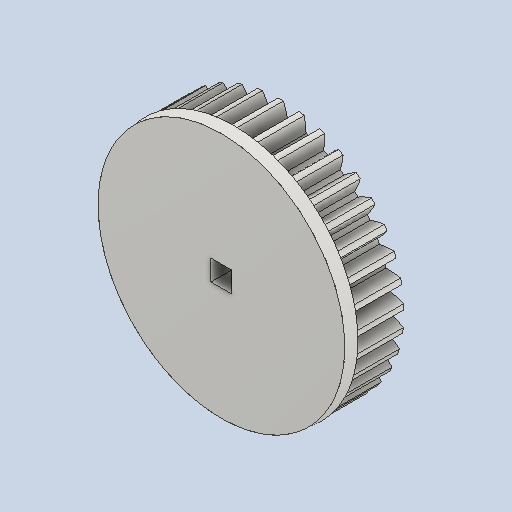
# Autodesk Inventor part: Spur Gear2
Saved by Autodesk Inventor 2022 (Build 260153000, 153)
## iProperties
CustomPartVersion: 1
Created: 2022-03-16
Part Number: Spur Gear2
Material: Steel
Document SubType Name: Modeling
Designer: zac-h
Categories: <?xml version="1.0" encoding="UTF-16"?> <MemberInstance><Categories><FamilyTemplate><FamilyTemplateParameter ValueType="xs:double" Id="1" ObjectReferenceKey="da_z" ObjectType="kUserParameterObject"/><FamilyTemplateParameter ValueType="xs:double" Id="2" ObjectReferenceKey="da_b" ObjectType="kUserParameterObject"/><FamilyTemplateParameter ValueType="xs:double" Id="3" ObjectReferenceKey="da_beta" ObjectType="kUserParameterObject"/><FamilyTemplateParameter ValueType="xs:double" Id="4" ObjectReferenceKey="da_da" ObjectType="kUserParameterObject"/><FamilyTemplateParameter ValueType="xs:double" Id="5" ObjectReferenceKey="da_aw" ObjectType="kUserParameterObject"/><FamilyTemplateParameter ValueType="xs:string" Id="6" ObjectReferenceKey="EAIAABAAAAC/AAAAAAAAAIAAAAAAAAAA" ObjectType="83910656" SubObjectId="SurfaceGeometry"/></FamilyTemplate><ParamToTemplateMap><ParamToTemplate CategoryParameter="//CategoryParameter[@InternalName='046C89C9-8512-4d59-83FE-43B91F4F132A']" TemplateParameter="1"/><ParamToTemplate CategoryParameter="//CategoryParameter[@InternalName='2552DF32-E462-4b46-AEBF-C6C7768E72AC']" TemplateParameter="2"/><ParamToTemplate CategoryParameter="//CategoryParameter[@InternalName='C9EE641D-15FC-4fae-A226-E94C4372FDD7']" TemplateParameter="3"/><ParamToTemplate><ParamToTemplate CategoryParameter="//CategoryParameter[@InternalName='00B6519A-459B-49c7-AD84-2E56D39A5744']" ConstantValue="0.273428"/></ParamToTemplate><ParamToTemplate><ParamToTemplate CategoryParameter="//CategoryParameter[@InternalName='04B31F0E-C7A6-4894-AA32-9629BEFACF47']" ConstantValue="1.000000"/></ParamToTemplate><ParamToTemplate><ParamToTemplate CategoryParameter="//CategoryParameter[@InternalName='43CBEC2E-7847-49e7-A936-2F7889FCB2D9']" ConstantValue="0.250000"/></ParamToTemplate><ParamToTemplate><ParamToTemplate CategoryParameter="//CategoryParameter[@InternalName='B1EFC894-105D-4ebd-86BF-FA20ED196853']" ConstantValue="0.333500"/></ParamToTemplate><ParamToTemplate><ParamToTemplate CategoryParameter="//CategoryParameter[@InternalName='51175063-3D10-4879-93E8-6246FE8B403D']" ConstantValue="2061532430.657340"/></ParamToTemplate><ParamToTemplate><ParamToTemplate CategoryParameter="//CategoryParameter[@InternalName='A3A52E27-4454-46a9-B0BD-C932399B70AF']" ConstantValue="0.300000"/></ParamToTemplate><ParamToTemplate><ParamToTemplate CategoryParameter="//CategoryParameter[@InternalName='91B76062-C214-41d9-B1B9-14D2AB99603D']" ConstantValue="0.100000"/></ParamToTemplate><ParamToTemplate><ParamToTemplate CategoryParameter="//CategoryParameter[@InternalName='374E806E-8B8A-4dda-A9AA-1039D6500AD2']" ConstantValue="10.000000"/></ParamToTemplate><ParamToTemplate><ParamToTemplate CategoryParameter="//CategoryParameter[@InternalName='2D373A89-B862-43d6-8D0B-0CBF12AB9F6C']" ConstantValue="0.253073"/></ParamToTemplate><ParamToTemplate CategoryParameter="//CategoryParameter[@InternalName='37777632-D6A2-4fac-9D53-DB8ACD95C989']" TemplateParameter="4"/><ParamToTemplate CategoryParameter="//CategoryParameter[@InternalName='FD1017F1-B727-4f7e-9707-0F86F1FF9423']" TemplateParameter="5"/><ParamToTemplate><ParamToTemplate CategoryParameter="//CategoryParameter[@InternalName='9E1B4470-B2D3-4ff1-B813-535BB4CDF51A']" ConstantValue="3523220.976809"/></ParamToTemplate><ParamToTemplate><ParamToTemplate CategoryParameter="//CategoryParameter[@InternalName='F8452263-BFF6-458c-9FB1-07C4B99E95CD']" ConstantValue="11397033.805607"/></ParamToTemplate><ParamToTemplate><ParamToTemplate CategoryParameter="//CategoryParameter[@InternalName='3E3BB259-FD49-497f-8171-6EBC954A3479']" ConstantValue="2.000000"/></ParamToTemplate><ParamToTemplate CategoryParameter="//CategoryParameter[@InternalName='27C3BAF2-7550-4e4b-AE2C-0DB134B7D9B7']" TemplateParameter="6"/></ParamToTemplateMap><Category DisplayName="Gear" InternalName="DC85795E-93AB-48d5-8EEE-5A27447B64BD" Mnemonic="Gear"><CategoryParameter DisplayName="z" InternalName="046C89C9-8512-4d59-83FE-43B91F4F132A" Mnemonic="z"/><CategoryParameter DisplayName="b" InternalName="2552DF32-E462-4b46-AEBF-C6C7768E72AC" Mnemonic="b"/><CategoryParameter DisplayName="||b|" InternalName="C9EE641D-15FC-4fae-A226-E94C4372FDD7" Mnemonic="beta"/><CategoryParameter DisplayName="x" InternalName="00B6519A-459B-49c7-AD84-2E56D39A5744" Mnemonic="x"/><CategoryParameter DisplayName="a*" InternalName="04B31F0E-C7A6-4894-AA32-9629BEFACF47" Mnemonic="a"/><CategoryParameter DisplayName="c*" InternalName="43CBEC2E-7847-49e7-A936-2F7889FCB2D9" Mnemonic="c"/><CategoryParameter DisplayName="r|.f|*" InternalName="B1EFC894-105D-4ebd-86BF-FA20ED196853" Mnemonic="rf"/><CategoryParameter DisplayName="E" InternalName="51175063-3D10-4879-93E8-6246FE8B403D" Mnemonic="E"/><CategoryParameter DisplayName="||m|" InternalName="A3A52E27-4454-46a9-B0BD-C932399B70AF" Mnemonic="mi"/><Category DisplayName="SpurGear" InternalName="26C5A22E-A91E-4dfd-A3B3-23CCAFAE1764" Mnemonic="SpurGear"><CategoryParameter DisplayName="m" InternalName="91B76062-C214-41d9-B1B9-14D2AB99603D" Mnemonic="m"/><CategoryParameter DisplayName="P" InternalName="374E806E-8B8A-4dda-A9AA-1039D6500AD2" Mnemonic="PP"/><CategoryParameter DisplayName="||a|" InternalName="2D373A89-B862-43d6-8D0B-0CBF12AB9F6C" Mnemonic="alpha"/><CategoryParameter DisplayName="d|.a|" InternalName="37777632-D6A2-4fac-9D53-DB8ACD95C989" Mnemonic="da"/><CategoryParameter DisplayName="a|.w|" InternalName="FD1017F1-B727-4f7e-9707-0F86F1FF9423" Mnemonic="aw"/><CategoryParameter DisplayName="||s||.Flim|" InternalName="9E1B4470-B2D3-4ff1-B813-535BB4CDF51A" Mnemonic="sFlim"/><CategoryParameter DisplayName="||s||.Hlim|" InternalName="F8452263-BFF6-458c-9FB1-07C4B99E95CD" Mnemonic="sHlim"/><CategoryParameter DisplayName="type" InternalName="3E3BB259-FD49-497f-8171-6EBC954A3479" Mnemonic="type"/><CategoryParameter DisplayName="PitchDiameter" InternalName="27C3BAF2-7550-4e4b-AE2C-0DB134B7D9B7" Mnemonic="IDS_PITCHDIAM"/></Category></Category></Categories></MemberInstance>
Density: 1 g/cm^3
Appearance: Steel
d9: 0.000 in
d14: 0.000 in
d15: 0.935 in
d16: 0.000 in
d17: 0.000 in
d18: 0.000 in
d19: 0.935 in
Author: zac-h
## iProperties of the stored document Spur Gear21_3DPrint.ipt
Created: 2022-03-19
Part Number: Spur Gear21_3DPrint
Material: Generic
Document SubType Name: Modeling
Designer: zac-h
Density: 1 g/cm^3
Appearance: Default
Author: zac-h
Autodesk Inventor part; units mm, degrees
sketch "Sketch1" plane through (0, 0, 0) normal (0, 0, 1) x (1, 0, 0)
  circle A0 centre (0, 0) radius 19.7541
  dimension "d0" = 39.5082
  constraints: 1 centre point
  measures "d0" diameter of A0
extrude "Extrusion1" add sketch "Sketch1" along normal blind 9.525
sketch "Sketch2" plane through (0, 0, 0) normal (0, 0, -1) x (-1, 0, 0)
  circle A0 centre (0, 0) radius 19.7541 projected
  circle A1 centre (0, 0) radius 18.5
  dimension "d3" = 37
  constraints: 1 centre point, 1 coincident
  measures "d3" diameter of A1
surface extrude "Pitch Diameter" sketch "Sketch2" against normal through all shown no curves A1
ref_plane "Work Plane1" through (0, 0, 0) normal (1, 0, 0) x (0, 1, 0)
ref_plane "Work Plane2" through (0, 0, 0) normal (0.9963975, 0.0848059, 0) x (0, 0, 1)
ref_plane "Work Plane3" through (0, 0, 4.7625) normal (0, 0, -1) x (-1, 0, 0)
spur gear teeth "Spur Gear" teeth 37 pitch diameter 37 tip diameter 39.5082 root diameter 35.0469 face width 9.525 start plane through (0, 0, 0) normal (0, 0, -1) x (-1, 0, 0)
sketch "Sketch3" plane through (0, 0, 9.525) normal (0, 0, 1) x (1, 0, 0)
  line L0 (-1.6625, 1.6625) -> (1.6625, 1.6625)
  line L1 (1.6625, 1.6625) -> (1.6625, -1.6625)
  line L2 (1.6625, -1.6625) -> (-1.6625, -1.6625)
  line L3 (-1.6625, -1.6625) -> (-1.6625, 1.6625)
  line L4 (-1.6625, 1.6625) -> (1.6625, -1.6625) construction
  line L5 (1.6625, 1.6625) -> (-1.6625, -1.6625) construction
  point P0 (0, 0)
  dimension "d20" = 3.325
  constraints: 12 end point, 2 midpoint, 2 parallel, 2 perpendicular, 1 horizontal
  measures "d20" distance of L1.end L2.end
extrude "Extrusion2" cut sketch "Sketch3" against normal through all
sketch "Sketch4" plane through (0, 0, 0) normal (0, 0, -1) x (-1, 0, 0)
  circle A0 centre (0, 0) radius 6.05
  line L0 (-1.6625, -1.6625) -> (-1.6625, 1.6625) projected
  line L1 (-1.6625, 1.6625) -> (1.6625, 1.6625) projected
  line L2 (1.6625, 1.6625) -> (1.6625, -1.6625) projected
  line L3 (1.6625, -1.6625) -> (-1.6625, -1.6625) projected
  arc A1 (4.0546, 17.0479) -> (3.751, 19.3947) centre (-6.6227, 16.8595) ccw projected
  arc A2 (3.751, 19.3947) -> (2.9244, 19.5364) centre (0, 0) ccw projected
  arc A3 (2.9244, 19.5364) -> (1.8564, 17.4248) centre (11.861, 13.6902) ccw projected
  arc A4 (1.8564, 17.4248) -> (1.1152, 17.4879) centre (0, 0) ccw projected
  arc A5 (1.1152, 17.4879) -> (0.4193, 19.7496) centre (-9.3767, 15.4978) ccw projected
  arc A6 (0.4193, 19.7496) -> (-0.4193, 19.7496) centre (0, 0) ccw projected
  arc A7 (-0.4193, 19.7496) -> (-1.1152, 17.4879) centre (9.3767, 15.4978) ccw projected
  arc A8 (-1.1152, 17.4879) -> (-1.8564, 17.4248) centre (0, 0) ccw projected
  arc A9 (-1.8564, 17.4248) -> (-2.9244, 19.5364) centre (-11.861, 13.6902) ccw projected
  arc A10 (-2.9244, 19.5364) -> (-3.751, 19.3947) centre (0, 0) ccw projected
  arc A11 (-3.751, 19.3947) -> (-4.0546, 17.0479) centre (6.6227, 16.8595) ccw projected
  arc A12 (-4.0546, 17.0479) -> (-4.7745, 16.8605) centre (0, 0) ccw projected
  arc A13 (-4.7745, 16.8605) -> (-6.1841, 18.7612) centre (-14.004, 11.4887) ccw projected
  arc A14 (-6.1841, 18.7612) -> (-6.9747, 18.4818) centre (0, 0) ccw projected
  arc A15 (-6.9747, 18.4818) -> (-6.8774, 16.1175) centre (3.6782, 17.7363) ccw projected
  arc A16 (-6.8774, 16.1175) -> (-7.5552, 15.811) centre (0, 0) ccw projected
  arc A17 (-7.5552, 15.811) -> (-9.2658, 17.4462) centre (-15.7442, 8.9568) ccw projected
  arc A18 (-9.2658, 17.4462) -> (-9.9978, 17.0372) centre (0, 0) ccw projected
  arc A19 (-9.9978, 17.0372) -> (-9.5023, 14.7233) centre (0.6278, 18.1028) ccw projected
  arc A20 (-9.5023, 14.7233) -> (-10.1186, 14.3068) centre (0, 0) ccw projected
  arc A21 (-10.1186, 14.3068) -> (-12.0809, 15.6293) centre (-17.0314, 6.1672) ccw projected
  arc A22 (-12.0809, 15.6293) -> (-12.7333, 15.1025) centre (0, 0) ccw projected
  arc A23 (-12.7333, 15.1025) -> (-11.8539, 12.9057) centre (-2.4406, 17.9485) ccw projected
  arc A24 (-11.8539, 12.9057) -> (-12.3909, 12.3909) centre (0, 0) ccw projected
  arc A25 (-12.3909, 12.3909) -> (-14.5485, 13.3628) centre (-17.8287, 3.2001) ccw projected
  arc A26 (-14.5485, 13.3628) -> (-15.1025, 12.7333) centre (0, 0) ccw projected
  arc A27 (-15.1025, 12.7333) -> (-13.8644, 10.7167) centre (-5.4388, 17.2778) ccw projected
  arc A28 (-13.8644, 10.7167) -> (-14.3068, 10.1186) centre (0, 0) ccw projected
  arc A29 (-14.3068, 10.1186) -> (-16.5975, 10.7119) centre (-18.1131, 0.141) ccw projected
  arc A30 (-16.5975, 10.7119) -> (-17.0372, 9.9978) centre (0, 0) ccw projected
  arc A31 (-17.0372, 9.9978) -> (-15.4761, 8.2195) centre (-8.2805, 16.1101) ccw projected
  arc A32 (-15.4761, 8.2195) -> (-15.811, 7.5552) centre (0, 0) ccw projected
  arc A33 (-15.811, 7.5552) -> (-18.1691, 7.7528) centre (-17.8764, -2.9221) ccw projected
  arc A34 (-18.1691, 7.7528) -> (-18.4818, 6.9747) centre (0, 0) ccw projected
  arc A35 (-18.4818, 6.9747) -> (-16.6426, 5.4857) centre (-10.884, 14.479) ccw projected
  arc A36 (-16.6426, 5.4857) -> (-16.8605, 4.7745) centre (0, 0) ccw projected
  arc A37 (-16.8605, 4.7745) -> (-19.218, 4.5707) centre (-17.1254, -5.9012) ccw projected
  arc A38 (-19.218, 4.5707) -> (-19.3947, 3.751) centre (0, 0) ccw projected
  arc A39 (-19.3947, 3.751) -> (-17.3303, 2.5942) centre (-13.1744, 12.4313) ccw projected
  arc A40 (-17.3303, 2.5942) -> (-17.4248, 1.8564) centre (0, 0) ccw projected
  arc A41 (-17.4248, 1.8564) -> (-19.714, 1.2571) centre (-15.8818, -8.7105) ccw projected
  arc A42 (-19.714, 1.2571) -> (-19.7496, 0.4193) centre (0, 0) ccw projected
  arc A43 (-19.7496, 0.4193) -> (-17.5195, -0.3719) centre (-15.0858, 10.026) ccw projected
  arc A44 (-17.5195, -0.3719) -> (-17.4879, -1.1152) centre (0, 0) ccw projected
  arc A45 (-17.4879, -1.1152) -> (-19.6429, -2.0927) centre (-14.1812, -11.2693) ccw projected
  arc A46 (-19.6429, -2.0927) -> (-19.5364, -2.9244) centre (0, 0) ccw projected
  arc A47 (-19.5364, -2.9244) -> (-17.2046, -3.3274) centre (-16.5633, 7.3323) ccw projected
  arc A48 (-17.2046, -3.3274) -> (-17.0479, -4.0546) centre (0, 0) ccw projected
  arc A49 (-17.0479, -4.0546) -> (-19.0067, -5.3822) centre (-12.0727, -13.5038) ccw projected
  arc A50 (-19.0067, -5.3822) -> (-18.7612, -6.1841) centre (0, 0) ccw projected
  arc A51 (-18.7612, -6.1841) -> (-16.3948, -6.1871) centre (-17.5642, 4.4276) ccw projected
  arc A52 (-16.3948, -6.1871) -> (-16.1175, -6.8774) centre (0, 0) ccw projected
  arc A53 (-16.1175, -6.8774) -> (-17.8237, -8.517) centre (-9.6169, -15.3499) ccw projected
  arc A54 (-17.8237, -8.517) -> (-17.4462, -9.2658) centre (0, 0) ccw projected
  arc A55 (-17.4462, -9.2658) -> (-15.1134, -8.8689) centre (-18.0598, 1.3956) ccw projected
  arc A56 (-15.1134, -8.8689) -> (-14.7233, -9.5023) centre (0, 0) ccw projected
  arc A57 (-14.7233, -9.5023) -> (-16.128, -11.4067) centre (-6.8844, -16.7543) ccw projected
  arc A58 (-16.128, -11.4067) -> (-15.6293, -12.0809) centre (0, 0) ccw projected
  arc A59 (-15.6293, -12.0809) -> (-13.3971, -11.2955) centre (-18.0359, -1.6766) ccw projected
  arc A60 (-13.3971, -11.2955) -> (-12.9057, -11.8539) centre (0, 0) ccw projected
  arc A61 (-12.9057, -11.8539) -> (-13.9682, -13.9682) centre (-3.9539, -17.6768) ccw projected
  arc A62 (-13.9682, -13.9682) -> (-13.3628, -14.5485) centre (0, 0) ccw projected
  arc A63 (-13.3628, -14.5485) -> (-11.2955, -13.3971) centre (-17.4931, -4.7006) ccw projected
  arc A64 (-11.2955, -13.3971) -> (-10.7167, -13.8644) centre (0, 0) ccw projected
  arc A65 (-10.7167, -13.8644) -> (-11.4067, -16.128) centre (-0.9097, -18.0908) ccw projected
  arc A66 (-11.4067, -16.128) -> (-10.7119, -16.5975) centre (0, 0) ccw projected
  arc A67 (-10.7119, -16.5975) -> (-8.8689, -15.1134) centre (-16.4471, -7.5893) ccw projected
  arc A68 (-8.8689, -15.1134) -> (-8.2195, -15.4761) centre (0, 0) ccw projected
  arc A69 (-8.2195, -15.4761) -> (-8.517, -17.8237) centre (2.1608, -17.9843) ccw projected
  arc A70 (-8.517, -17.8237) -> (-7.7528, -18.1691) centre (0, 0) ccw projected
  arc A71 (-7.7528, -18.1691) -> (-6.1871, -16.3948) centre (-14.9279, -10.2597) ccw projected
  arc A72 (-6.1871, -16.3948) -> (-5.4857, -16.6426) centre (0, 0) ccw projected
  arc A73 (-5.4857, -16.6426) -> (-5.3822, -19.0067) centre (5.1691, -17.3604) ccw projected
  arc A74 (-5.3822, -19.0067) -> (-4.5707, -19.218) centre (0, 0) ccw projected
  arc A75 (-4.5707, -19.218) -> (-3.3274, -17.2046) centre (-12.9793, -12.635) ccw projected
  arc A76 (-3.3274, -17.2046) -> (-2.5942, -17.3303) centre (0, 0) ccw projected
  arc A77 (-2.5942, -17.3303) -> (-2.0927, -19.6429) centre (8.0286, -16.2371) ccw projected
  arc A78 (-2.0927, -19.6429) -> (-1.2571, -19.714) centre (0, 0) ccw projected
  arc A79 (-1.2571, -19.714) -> (-0.3719, -17.5195) centre (-10.6572, -14.6467) ccw projected
  arc A80 (-0.3719, -17.5195) -> (0.3719, -17.5195) centre (0, 0) ccw projected
  arc A81 (0.3719, -17.5195) -> (1.2571, -19.714) centre (10.6572, -14.6467) ccw projected
  arc A82 (1.2571, -19.714) -> (2.0927, -19.6429) centre (0, 0) ccw projected
  arc A83 (2.0927, -19.6429) -> (2.5942, -17.3303) centre (-8.0286, -16.2371) ccw projected
  arc A84 (2.5942, -17.3303) -> (3.3274, -17.2046) centre (0, 0) ccw projected
  arc A85 (3.3274, -17.2046) -> (4.5707, -19.218) centre (12.9793, -12.635) ccw projected
  arc A86 (4.5707, -19.218) -> (5.3822, -19.0067) centre (0, 0) ccw projected
  arc A87 (5.3822, -19.0067) -> (5.4857, -16.6426) centre (-5.1691, -17.3604) ccw projected
  arc A88 (5.4857, -16.6426) -> (6.1871, -16.3948) centre (0, 0) ccw projected
  arc A89 (6.1871, -16.3948) -> (7.7528, -18.1691) centre (14.9279, -10.2597) ccw projected
  arc A90 (7.7528, -18.1691) -> (8.517, -17.8237) centre (0, 0) ccw projected
  arc A91 (8.517, -17.8237) -> (8.2195, -15.4761) centre (-2.1608, -17.9843) ccw projected
  arc A92 (8.2195, -15.4761) -> (8.8689, -15.1134) centre (0, 0) ccw projected
  arc A93 (8.8689, -15.1134) -> (10.7119, -16.5975) centre (16.4471, -7.5893) ccw projected
  arc A94 (10.7119, -16.5975) -> (11.4067, -16.128) centre (0, 0) ccw projected
  arc A95 (11.4067, -16.128) -> (10.7167, -13.8644) centre (0.9097, -18.0908) ccw projected
  arc A96 (10.7167, -13.8644) -> (11.2955, -13.3971) centre (0, 0) ccw projected
  arc A97 (11.2955, -13.3971) -> (13.3628, -14.5485) centre (17.4931, -4.7006) ccw projected
  arc A98 (13.3628, -14.5485) -> (13.9682, -13.9682) centre (0, 0) ccw projected
  arc A99 (13.9682, -13.9682) -> (12.9057, -11.8539) centre (3.9539, -17.6768) ccw projected
  arc A100 (12.9057, -11.8539) -> (13.3971, -11.2955) centre (0, 0) ccw projected
  arc A101 (13.3971, -11.2955) -> (15.6293, -12.0809) centre (18.0359, -1.6766) ccw projected
  arc A102 (15.6293, -12.0809) -> (16.128, -11.4067) centre (0, 0) ccw projected
  arc A103 (16.128, -11.4067) -> (14.7233, -9.5023) centre (6.8844, -16.7543) ccw projected
  arc A104 (14.7233, -9.5023) -> (15.1134, -8.8689) centre (0, 0) ccw projected
  arc A105 (15.1134, -8.8689) -> (17.4462, -9.2658) centre (18.0598, 1.3956) ccw projected
  arc A106 (17.4462, -9.2658) -> (17.8237, -8.517) centre (0, 0) ccw projected
  arc A107 (17.8237, -8.517) -> (16.1175, -6.8774) centre (9.6169, -15.3499) ccw projected
  arc A108 (16.1175, -6.8774) -> (16.3948, -6.1871) centre (0, 0) ccw projected
  arc A109 (16.3948, -6.1871) -> (18.7612, -6.1841) centre (17.5642, 4.4276) ccw projected
  arc A110 (18.7612, -6.1841) -> (19.0067, -5.3822) centre (0, 0) ccw projected
  arc A111 (19.0067, -5.3822) -> (17.0479, -4.0546) centre (12.0727, -13.5038) ccw projected
  arc A112 (17.0479, -4.0546) -> (17.2046, -3.3274) centre (0, 0) ccw projected
  arc A113 (17.2046, -3.3274) -> (19.5364, -2.9244) centre (16.5633, 7.3323) ccw projected
  arc A114 (19.5364, -2.9244) -> (19.6429, -2.0927) centre (0, 0) ccw projected
  arc A115 (19.6429, -2.0927) -> (17.4879, -1.1152) centre (14.1812, -11.2693) ccw projected
  arc A116 (17.4879, -1.1152) -> (17.5195, -0.3719) centre (0, 0) ccw projected
  arc A117 (17.5195, -0.3719) -> (19.7496, 0.4193) centre (15.0858, 10.026) ccw projected
  arc A118 (19.7496, 0.4193) -> (19.714, 1.2571) centre (0, 0) ccw projected
  arc A119 (19.714, 1.2571) -> (17.4248, 1.8564) centre (15.8818, -8.7105) ccw projected
  arc A120 (17.4248, 1.8564) -> (17.3303, 2.5942) centre (0, 0) ccw projected
  arc A121 (17.3303, 2.5942) -> (19.3947, 3.751) centre (13.1744, 12.4313) ccw projected
  arc A122 (19.3947, 3.751) -> (19.218, 4.5707) centre (0, 0) ccw projected
  arc A123 (19.218, 4.5707) -> (16.8605, 4.7745) centre (17.1254, -5.9012) ccw projected
  arc A124 (16.8605, 4.7745) -> (16.6426, 5.4857) centre (0, 0) ccw projected
  arc A125 (16.6426, 5.4857) -> (18.4818, 6.9747) centre (10.884, 14.479) ccw projected
  arc A126 (18.4818, 6.9747) -> (18.1691, 7.7528) centre (0, 0) ccw projected
  arc A127 (18.1691, 7.7528) -> (15.811, 7.5552) centre (17.8764, -2.9221) ccw projected
  arc A128 (15.811, 7.5552) -> (15.4761, 8.2195) centre (0, 0) ccw projected
  arc A129 (15.4761, 8.2195) -> (17.0372, 9.9978) centre (8.2805, 16.1101) ccw projected
  arc A130 (17.0372, 9.9978) -> (16.5975, 10.7119) centre (0, 0) ccw projected
  arc A131 (16.5975, 10.7119) -> (14.3068, 10.1186) centre (18.1131, 0.141) ccw projected
  arc A132 (14.3068, 10.1186) -> (13.8644, 10.7167) centre (0, 0) ccw projected
  arc A133 (13.8644, 10.7167) -> (15.1025, 12.7333) centre (5.4388, 17.2778) ccw projected
  arc A134 (15.1025, 12.7333) -> (14.5485, 13.3628) centre (0, 0) ccw projected
  arc A135 (14.5485, 13.3628) -> (12.3909, 12.3909) centre (17.8287, 3.2001) ccw projected
  arc A136 (12.3909, 12.3909) -> (11.8539, 12.9057) centre (0, 0) ccw projected
  arc A137 (11.8539, 12.9057) -> (12.7333, 15.1025) centre (2.4406, 17.9485) ccw projected
  arc A138 (12.7333, 15.1025) -> (12.0809, 15.6293) centre (0, 0) ccw projected
  arc A139 (12.0809, 15.6293) -> (10.1186, 14.3068) centre (17.0314, 6.1672) ccw projected
  arc A140 (10.1186, 14.3068) -> (9.5023, 14.7233) centre (0, 0) ccw projected
  arc A141 (9.5023, 14.7233) -> (9.9978, 17.0372) centre (-0.6278, 18.1028) ccw projected
  arc A142 (9.9978, 17.0372) -> (9.2658, 17.4462) centre (0, 0) ccw projected
  arc A143 (9.2658, 17.4462) -> (7.5552, 15.811) centre (15.7442, 8.9568) ccw projected
  arc A144 (7.5552, 15.811) -> (6.8774, 16.1175) centre (0, 0) ccw projected
  arc A145 (6.8774, 16.1175) -> (6.9747, 18.4818) centre (-3.6782, 17.7363) ccw projected
  arc A146 (6.9747, 18.4818) -> (6.1841, 18.7612) centre (0, 0) ccw projected
  arc A147 (6.1841, 18.7612) -> (4.7745, 16.8605) centre (14.004, 11.4887) ccw projected
  arc A148 (4.7745, 16.8605) -> (4.0546, 17.0479) centre (0, 0) ccw projected
  dimension "d23" = 12.1
  constraints: 1 centre point, 1 coincident
  measures "d23" diameter of A0
extrude "Extrusion3" add sketch "Sketch4" along normal blind 1.5875 contours A0
chamfer "Chamfer1" distance 1.5875 angle 45 1 edges at (6.05, 0, 0)
sketch "Sketch5" plane through (0, 0, 0) normal (1, 0, 0) x (0, 1, 0)
  line L0 (-17.5, 0) -> (17.5, 0)
  line L1 (17.5, 0) -> (17.5, 6.35)
  line L2 (17.5, 6.35) -> (-17.5, 6.35)
  line L3 (-17.5, 6.35) -> (-17.5, 0)
  line L4 (19.9228, 7.55) -> (19.75, 9.525)
  line L5 (19.75, 9.525) -> (0, 9.525)
  line L6 (0, 9.525) -> (0, 0)
  line L7 (17.5, 6.35) -> (17.5, 7.55)
  line L8 (17.5, 7.55) -> (19.9228, 7.55)
  line L9 (17.5465, 7.55) -> (17.5465, 9.525)
  line L10 (16.7129, 9.525) -> (17.5, 6.35)
  point P0 (0, 6.35)
  dimension "d29" = 35
  dimension "d30" = 6.35
  dimension "d32" = 9.525
  dimension "d33" = 39.5
  dimension "d35" = 1.2
  dimension "d36" = 85
  constraints: 22 end point, 3 perpendicular, 3 point on line, 2 parallel, 2 vertical, 1 coincident, 1 horizontal, 1 midpoint
  measures "d29" distance of L2.end L1.end
  measures "d30" distance of L1.end L0.end
  measures "d32" distance between parallel lines of L0 L5
  measures "d33" diameter of L4.end L6
  measures "d35" distance from line of L1.end L8
  measures "d36" angle of L4 L8
revolve "Revolution1" add sketch "Sketch5" angle 360 about axis through (0, 0, 9.525) along (0, 0, -1) contours L10 L5 L9 L8 L7 | L9 L5 L4 L8
equation "\"d0\" = da_da"
equation "\"d1\" = da_b"
equation "\"d3\" = da_d"
equation "\"d15\" = da_aw"
equation "\"d19\" = da_aw"
equation "\"da_da\" = 39.50816"
equation "\"da_b\" = 9.525"
equation "\"da_d\" = 37"
equation "\"da_aw\" = 23.75408"
body "Solid1"
body "Srf1"
